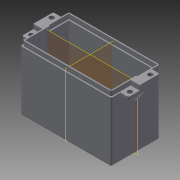
# Autodesk Inventor part: sensor1_3t
Saved by Autodesk Inventor 2015 (Build 190159000, 159)
## iProperties
Created: 2015-12-11
Part Number: sensor1_3t
Material: Generic
Document SubType Name: Modeling
Designer: mca20
Density: 1 g/cm^3
Appearance: Default
Author: mca20
Autodesk Inventor part; units mm, degrees
ref_plane "YZ Plane" through (0, 0, 0) normal (1, 0, 0) x (0, 1, 0)
ref_plane "XZ Plane" through (0, 0, 0) normal (0, 1, 0) x (-1, 0, 0)
ref_plane "XY Plane" through (0, 0, 0) normal (0, 0, 1) x (1, 0, 0)
sketch "Sketch3" plane through (0, 0, 0) normal (0, 1, 0) x (-1, 0, 0)
  line L0 (0, 0) -> (-55, 0)
  line L1 (-55, 0) -> (-55, -35.25)
  line L2 (-55, -35.25) -> (0, -35.25)
  line L3 (0, -35.25) -> (0, 0)
  line L4 (1.5, 1.5) -> (-56.5, 1.5)
  line L5 (-56.5, 1.5) -> (-56.5, -36.75)
  line L6 (-56.5, -36.75) -> (1.5, -36.75)
  line L7 (1.5, -36.75) -> (1.5, 1.5)
  dimension "d0" = 35.25
  dimension "d1" = 55
  dimension "d4" = 38.25
  dimension "d5" = 58
  dimension "d6" = 1.5
  dimension "d7" = 1.5
  constraints: 16 end point, 4 parallel, 2 horizontal, 2 perpendicular
  measures "d0" distance between parallel lines of L2 L0
  measures "d1" distance between parallel lines of L1 L3
  measures "d4" distance between parallel lines of L6 L4
  measures "d5" distance between parallel lines of L5 L7
  measures "d6" distance between parallel lines of L5 L1
  measures "d7" distance between parallel lines of L0 L4
extrude "Extrusion1" add sketch "Sketch3" against normal blind 1.5 contours L3 L2 L1 L0 | L7 L6 L5 L4
sketch "Sketch5" plane through (0, 0, 0) normal (0, 1, 0) x (-1, 0, 0)
  line L0 (-55, 0) -> (-55, -35.25)
  line L1 (-55, -35.25) -> (0, -35.25)
  line L2 (0, -35.25) -> (0, 0)
  line L3 (-56.5, 1.5) -> (-56.5, -36.75)
  line L4 (-56.5, -36.75) -> (1.5, -36.75)
  line L5 (1.5, -36.75) -> (1.5, 1.5)
  line L6 (0, 0) -> (0, 1.5)
  line L7 (1.5, 1.5) -> (0, 1.5)
  line L8 (-55, 0) -> (-55, 1.5)
  line L9 (-55, 1.5) -> (-56.5, 1.5)
  dimension "d9" = 55
  dimension "d11" = 58
  dimension "d12" = 1.5
  constraints: 20 end point, 2 parallel, 1 perpendicular, 1 vertical
  measures "d9" distance between parallel lines of L0 L2
  measures "d11" distance between parallel lines of L3 L5
  measures "d12" distance between parallel lines of L3 L0
extrude "Extrusion2" add sketch "Sketch5" along normal blind 28
sketch "Sketch6" plane through (0, 28, 0) normal (0, 1, 0) x (1, 0, 0)
  line L0 (-1.5, -1.5) -> (56.5, -1.5)
  line L1 (56.5, -1.5) -> (56.5, 36.75)
  line L2 (56.5, 36.75) -> (-1.5, 36.75)
  line L3 (-1.5, 36.75) -> (-1.5, -1.5)
  point P0 (0, 0)
  constraints: 8 end point, 2 parallel, 1 horizontal, 1 perpendicular
extrude "Extrusion3" add sketch "Sketch6" along normal blind 1.5
sketch "Sketch7" plane through (0, 0, 1.5) normal (1, 0, 0) x (0, 0, -1)
  line L0 (8.375, 4.5) -> (23.375, 4.5)
  line L1 (23.375, 4.5) -> (23.375, 5.5)
  line L2 (23.375, 5.5) -> (8.375, 5.5)
  line L3 (8.375, 5.5) -> (8.375, 4.5)
  line L4 (36.75, 0) -> (36.75, 28) projected
  line L5 (0, 0) -> (0, 28) projected
  line L6 (36.75, 0) -> (0, 0) projected
  point P0 (1.5, 0)
  dimension "d20" = 15
  dimension "d21" = 1
  dimension "d22" = 13.375
  dimension "d23" = 8.375
  dimension "d40" = 4.5
  constraints: 8 end point, 2 parallel, 1 horizontal, 1 perpendicular
  measures "d20" distance from line of L1.end L3
  measures "d21" distance between parallel lines of L0 L2
  measures "d22" distance between parallel lines of L4 L1
  measures "d23" distance between parallel lines of L5 L3
  measures "d40" distance between parallel lines of L0 L6
ref_plane "Work Plane1" through (27.5, 0, 1.5) normal (1, 0, 0) x (0, 0, -1)
extrude "Extrusion4" add sketch "Sketch7" along normal blind 1
mirror "Mirror1" about plane through (27.5, 0, 1.5) normal (1, 0, 0) of "Extrusion4"
sketch "Sketch8" plane through (-1.5, -1.5, 1.5) normal (0, 0, 1) x (1, 0, 0)
  line L0 (0.75, 30.25) -> (57.25, 30.25)
  line L1 (57.25, 30.25) -> (57.25, 13.25)
  line L2 (0.75, 13.25) -> (0.75, 30.25)
  line L3 (0, 31) -> (58, 31) projected
  line L4 (0.75, 13.25) -> (0, 13.25)
  line L5 (57.25, 13.25) -> (58, 13.25)
  line L6 (0, 31) -> (0, 13.25)
  line L7 (0, 31) -> (0, 0) projected
  line L8 (58, 31) -> (58, 13.25)
  line L9 (58, 0) -> (58, 31) projected
  point P0 (1.5, 1.5)
  dimension "d27" = 0.75
  dimension "d29" = 56.5
  dimension "d31" = 17
  dimension "d65" = 0.75
  dimension "d84" = 17
  constraints: 14 end point, 2 collinear, 2 horizontal, 1 parallel, 1 perpendicular
  measures "d27" distance between parallel lines of L3 L0
  measures "d29" distance between parallel lines of L1 L2
  measures "d31" distance from line of L5.end L0
  measures "d65" distance between parallel lines of L2 L6
  measures "d84" distance between parallel lines of L4 L0
extrude "Extrusion5" add sketch "Sketch8" along normal blind 3
sketch "Sketch9" plane through (-1.5, -1.5, 1.5) normal (0, 0, 1) x (1, 0, 0)
  line L0 (0.75, 0.75) -> (57.25, 0.75)
  line L1 (57.25, 0.75) -> (57.25, 17.5)
  line L2 (0.75, 17.5) -> (0.75, 0.75)
  line L3 (1.5, 1.5) -> (56.5, 1.5) projected
  line L4 (57.25, 17.5) -> (56.5, 17.5)
  line L5 (56.5, 1.5) -> (56.5, 29.5) projected
  line L6 (56.5, 1.5) -> (56.5, 17.5)
  line L7 (56.5, 1.5) -> (1.5, 1.5)
  line L8 (0.75, 17.5) -> (1.5, 17.5)
  line L9 (1.5, 1.5) -> (1.5, 29.5) projected
  line L10 (1.5, 17.5) -> (1.5, 1.5)
  line L11 (1.5, 29.5) -> (56.5, 29.5) projected
  dimension "d34" = 0.75
  dimension "d36" = 56.5
  dimension "d69" = 16.75
  dimension "d70" = 16.75
  dimension "d97" = 28.75
  constraints: 16 end point, 4 horizontal, 2 collinear, 2 point on line, 1 parallel, 1 perpendicular
  measures "d34" distance between parallel lines of L3 L0
  measures "d36" distance between parallel lines of L1 L2
  measures "d69" distance between parallel lines of L0 L8
  measures "d70" distance between parallel lines of L0 L4
  measures "d97" distance between parallel lines of L11 L0
extrude "Extrusion6" add sketch "Sketch9" along normal blind 3 contours L2 L8 L9 L3 L5 L4 L1 L0
sketch "Sketch10" plane through (0, 0, -35.25) normal (0, 0, 1) x (1, 0, 0)
  line L0 (55, 0) -> (0, 0) projected
  line L1 (20.5, 0) -> (34.5, 0)
  line L2 (34.5, 0) -> (34.5, 3.3)
  line L3 (34.5, 3.3) -> (20.5, 3.3)
  line L4 (20.5, 3.3) -> (20.5, 0)
  line L5 (0, 0) -> (0, 28) projected
  dimension "d41" = 14
  dimension "d42" = 20.5
  dimension "d43" = 3.3
  constraints: 8 end point, 2 parallel, 1 horizontal, 1 perpendicular, 1 point on line
  measures "d41" distance between parallel lines of L2 L4
  measures "d42" distance between parallel lines of L5 L4
  measures "d43" distance between parallel lines of L0 L3
extrude "Extrusion7" add sketch "Sketch10" along normal blind 5
fillet "Fillet1" radius 1 8 edges at (56.5, 29.5, -16.125) (56.5, -1.5, -17.625) (56.5, 14, -36.75) (27.5, 29.5, -36.75) (27.5, -1.5, -36.75) (-1.5, 14, -36.75) (-1.5, 29.5, -16.125) (-1.5, -1.5, -17.625)
sketch "Sketch11" plane through (0, 28, -35.25) normal (0, 0, 1) x (1, 0, 0)
  circle A0 centre (27.5, -17.2) radius 4.95
  line L0 (20.5, -24.7) -> (34.5, -24.7) projected
  line L1 (0, -28) -> (0, 0) projected
  dimension "d47" = 9.9
  dimension "d48" = 7.5
  dimension "d49" = 27.5
  constraints: 1 centre point
  measures "d47" diameter of A0
  measures "d48" distance from line of L0 A0.centre
  measures "d49" distance from line of A0.centre L1
extrude "Extrusion8" cut sketch "Sketch11" against normal blind 5
fillet "Fillet2" radius 1 1 edges at (-0.75, -0.75, 3)
fillet "Fillet3" radius 1 1 edges at (55.75, -0.75, 3)
sketch "Sketch15" plane through (56.5, 11.75, 4.5) normal (1, 0, 0) x (0, 0, -1)
  line L0 (0, 0) -> (5, 0)
  line L1 (5, 0) -> (5, 12.75)
  line L2 (5, 12.75) -> (0, 12.75)
  line L3 (0, 12.75) -> (0, 0)
  line L4 (5, 0) -> (3, 0)
  line L5 (3, 0) -> (3, -7.25)
  line L6 (3, -7.25) -> (5, -7.25)
  line L7 (5, -7.25) -> (5, 0)
  point P0 (4.5, -11.75)
  point P1 (0, 4.25)
  point P2 (0, 17.75)
  dimension "d78" = 5
  dimension "d79" = 12.75
  dimension "d80" = 2
  dimension "d81" = 7.25
  dimension "d98" = 11.5
  dimension "d99" = 20
  dimension "d100" = 12.75
  dimension "d101" = 5
  constraints: 16 end point, 4 parallel, 2 horizontal, 2 perpendicular
  measures "d78" distance of L2.end L1.end
  measures "d79" distance of L1.end L0.end
  measures "d80" distance of L6.end L5.end
  measures "d81" distance of L5.end L4.end
  measures "d98" distance from line of L6 point (0, 4.25)
  measures "d99" distance between parallel lines of L6 L2
  measures "d100" distance between parallel lines of L0 L2
  measures "d101" distance from line of L2 point (0, 17.75)
extrude "Extrusion10" add sketch "Sketch15" along normal blind 5
mirror "Mirror3" about plane through (27.5, 0, 1.5) normal (1, 0, 0) of "Extrusion10"
fillet "Fillet7" radius 1 2 edges at (61.5, 24.5, 2) (61.5, 4.5, 0.5)
fillet "Fillet8" radius 1 2 edges at (-6.5, 24.5, 2) (-6.5, 4.5, 0.5)
sketch "Sketch16" plane through (-1.5, -1.5, 4.5) normal (0, 0, 1) x (1, 0, 0)
  circle A0 centre (60.5, 22.5) radius 1.5
  line L0 (63, 25) -> (63, 13.25) projected
  line L1 (58, 26) -> (62, 26) projected
  point P0 (1.5, 1.5)
  dimension "d87" = 3
  dimension "d88" = 2.5
  dimension "d89" = 3.5
  constraints: 1 centre point
  measures "d87" diameter of A0
  measures "d88" distance from line of L0 A0.centre
  measures "d89" distance from line of L1 A0.centre
extrude "Extrusion11" cut sketch "Sketch16" against normal blind 5
sketch "Sketch17" plane through (-0.5, -1.5, 1.5) normal (0, 0, 1) x (1, 0, 0)
  circle A0 centre (59.5, 9.5) radius 1.5
  line L0 (57, 6) -> (61, 6) projected
  line L1 (62, 7) -> (62, 25) projected
  point P0 (0.5, 1.5)
  dimension "d92" = 3
  dimension "d93" = 3.5
  dimension "d94" = 2.5
  constraints: 1 centre point
  measures "d92" diameter of A0
  measures "d93" distance from line of L0 A0.centre
  measures "d94" distance from line of L1 A0.centre
extrude "Extrusion12" cut sketch "Sketch17" against normal blind 2
mirror "Mirror4" about plane through (27.5, 0, 1.5) normal (1, 0, 0) of "Extrusion11", "Extrusion12"
ref_plane "Work Plane5" through (0, 14, 0) normal (0, -1, 0) x (1, 0, 0)
sketch "Sketch18" plane through (0, 14, 0) normal (0, -1, 0) x (1, 0, 0)
  line L0 (61.5, -0.5) -> (65.4816, -0.5) construction
  line L1 (61.5, -0.5) -> (59.7504, -2.9987)
  line L2 (61.5, -0.5) -> (64.5503, -0.5) construction
  point P0 (0, 0)
  dimension "d104" = 125
  constraints: 6 end point, 2 horizontal, 1 equal length
  measures "d104" angle of L1 L2
extrude "Rib1" add sketch "Sketch18" along normal mid plane 2 rib yes fills toward (60.5842, -1.7207) open curves L1
mirror "Mirror5" about plane through (27.5, 0, 1.5) normal (1, 0, 0) of "Rib1"
ref_plane "Work Plane7" through (0, 5, -6.875) normal (0, 1, 0) x (1, 0, 0)
sketch "Sketch20" plane through (0, 0, -35.25) normal (1, 0, 0) x (0, 0, -1)
  point P0 (-35.25, 0)
sketch "Sketch21" plane through (0, 5, -6.875) normal (0, 1, 0) x (1, 0, 0)
  line L0 (1, 15) -> (0.3662, 15.6338)
  line L1 (1, 15) -> (1.8964, 15) construction
  point P0 (0, -6.875)
  dimension "d120" = 135
  constraints: 4 end point, 1 equal length, 1 horizontal
  measures "d120" angle of L1 L0
extrude "Rib3" add sketch "Sketch21" along normal mid plane 1 rib yes fills toward (0.6477, 15.2816) open curves L0
mirror "Mirror7" about plane through (27.5, 0, 1.5) normal (1, 0, 0) of "Rib3"
equation "\"d7\" = d6"
equation "\"d31\" = d66"
equation "\"d70\" = d69"
equation "\"d66\" = 17"
body "Solid1"
